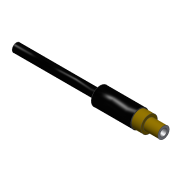
# Autodesk Inventor part: mmcx_coax_tip
Saved by Autodesk Inventor 2014 SP1 (Build 180222100, 222)
## iProperties
Created: 2014-03-24
Part Number: mmcx_coax_tip
Document SubType Name: Modeling
Designer: Robert Davis
Density: 1 g/cm^3
Material: Generic
Appearance: Default
Author: Robert Davis
Autodesk Inventor part; units mm, degrees
ref_plane "XZ Plane" through (0, 0, 0) normal (0, 1, 0) x (-1, 0, 0)
sketch "Sketch2" plane through (0, 0, 0) normal (0, 1, 0) x (-1, 0, 0)
  line L0 (0, 0) -> (-5, 0)
  line L1 (-5, 0) -> (-10, 1.6)
  line L2 (-10, 1.6) -> (-15, 1.6)
  dimension "d0" = 1.6
  dimension "d1" = 5
  dimension "d2" = 5
  dimension "d3" = 5
  constraints: 6 end point, 2 horizontal, 1 coincident
  measures "d0" distance between parallel lines of L0 L2
  measures "d1" distance of L0.start L0.end
  measures "d2" horizontal distance of L0.end L1.end
  measures "d3" distance of L1.end L2.end
sketch "Sketch3" plane through (0, 0, 0) normal (1, 0, 0) x (0, 1, 0)
  circle A0 centre (0, 0) radius 0.9
  dimension "d4" = 1.8
  constraints: 1 centre point, 1 coincident
  measures "d4" diameter of A0
sweep "Sweep1" [suppressed]
ref_plane "Work Plane1" through (0, 0, 1.6) normal (0, 0, 1) x (1, 0, 0)
sketch "Sketch4" plane through (0, 0, 1.6) normal (0, 0, 1) x (1, 0, 0)
  line L0 (25, -15) -> (25, -66.3933)
  line L1 (0, 0) -> (10, 0)
  arc A0 (25, -15) -> (10, 0) centre (10, -15) ccw
  dimension "d33" = 15
  dimension "d34" = 25
  dimension "d35" = 51.3933
  constraints: 4 end point, 2 point on circle, 2 tangent, 1 centre point, 1 perpendicular, 1 vertical
  measures "d33" radius of A0
  measures "d34" distance from line of L0 L1.start
  measures "d35" distance of L0.start L0.end
ref_plane "Work Plane2" through (15, 0, 0) normal (1, 0, 0) x (0, 1, 0)
sketch "Sketch5" plane through (15, 0, 0) normal (1, 0, 0) x (0, 1, 0)
  circle A0 centre (0, 1.6) radius 0.9
  point P0 (0, 0)
  dimension "d16" = 1.6
  dimension "d17" = 1.8
  constraints: 1 centre point, 1 vertical alignment
  measures "d16" distance of point (0, 0) A0.centre
  measures "d17" diameter of A0
sweep "Sweep2" [suppressed]
sketch "Sketch7" plane through (0, 0, 0) normal (1, 0, 0) x (0, 1, 0)
  circle A0 centre (0, 0) radius 0.75
  circle A1 centre (0, 0) radius 1.2065
  dimension "d21" = 2.413
  dimension "d36" = 1.5
  constraints: 3 coincident, 2 centre point
  measures "d21" diameter of A1
  measures "d36" diameter of A0
extrude "Extrusion1" add sketch "Sketch7" against normal blind 3.048
sketch "Sketch8" plane through (-3.048, 0, 0) normal (-1, 0, 0) x (0, 0, 1)
  circle A0 centre (0, 0) radius 0.9 projected
  circle A1 centre (0, 0) radius 1.2065 projected
  circle A2 centre (0, 0) radius 1.7526
  dimension "d24" = 3.5052
  constraints: 1 centre point, 1 coincident
  measures "d24" diameter of A2
extrude "Extrusion2" add sketch "Sketch8" along normal blind 2.032 contours A1 | A2
sketch "Sketch9" plane through (-5.08, 0, 0) normal (-1, 0, 0) x (0, 0, 1)
  circle A0 centre (0, 0) radius 0.9 projected
  circle A1 centre (0, 0) radius 1.7526 projected
  circle A2 centre (0, 0) radius 1.905
  dimension "d27" = 3.81
  constraints: 1 centre point, 1 coincident
  measures "d27" diameter of A2
extrude "Extrusion3" add sketch "Sketch9" along normal blind 8.382 contours A1 | A2
sketch "Sketch10" plane through (-13.462, 0, 0) normal (-1, 0, 0) x (0, 0, 1)
  circle A0 centre (0, 0) radius 0.9 projected
  circle A1 centre (0, 0) radius 1.905 projected
  circle A2 centre (0, 0) radius 0.9144
  dimension "d30" = 1.8288
  constraints: 1 centre point, 1 coincident
  measures "d30" diameter of A2
extrude "Extr_RG-178_72mils" add sketch "Sketch10" along normal blind 17.78 contours A2
body "Solid1"
